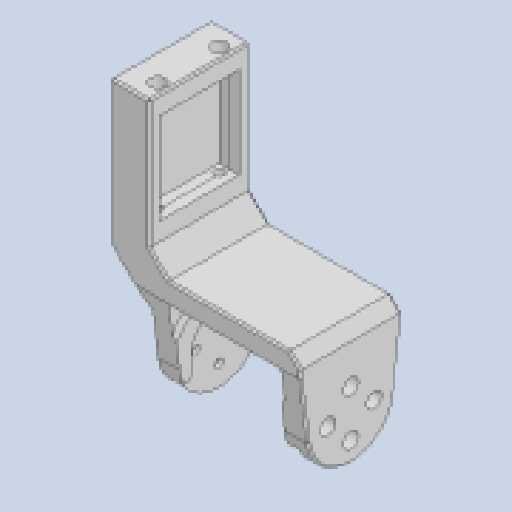
# Autodesk Inventor part: M-WristFlexion
Saved by Autodesk Inventor 2026 (Build 300175050, 175E)
## iProperties
Created: 2025-12-22
Part Number: M-WristFlexion
Material: Genérico
Document SubType Name: Modeling
Designer: user
Density: 1 g/cm^3
Appearance: Valor por defecto
Mass: 17.8828 g
Surface Area: 77.4828 cm^2
Volume: 17.8828 cm^3
Author: user
Autodesk Inventor part; units mm, degrees
ref_plane "YZ Plane" through (0, 0, 0) normal (1, 0, 0) x (0, 1, 0)
ref_plane "XZ Plane" through (0, 0, 0) normal (0, 1, 0) x (-1, 0, 0)
sketch "Boceto1" plane through (0, 0, 0) normal (0, 0, 1) x (1, 0, 0)
  line L0 (-14.6, -0.5214) -> (16.6711, -0.5214)
  line L1 (14.6, -5.5214) -> (-14.6, -5.5214)
  line L2 (14.6, -5.5214) -> (14.6, -32.4765)
  line L3 (14.6, -32.4765) -> (19.6, -32.4765)
  line L4 (19.6, -32.4765) -> (19.6, -3.4504)
  line L5 (-14.6, -5.5214) -> (-14.6, -32.4765)
  line L6 (-14.6, -32.4765) -> (-19.6, -32.4765)
  line L7 (-19.6, -32.4765) -> (-19.6, -9.6636)
  line L8 (-24.6, 9.3786) -> (-24.6, 32.5786)
  line L9 (-29.6, 37.5786) -> (-29.6, 0.3364)
  line L10 (-29.6, 0.3364) -> (-19.6, -9.6636)
  line L11 (16.6711, -0.5214) -> (19.6, -3.4504)
  line L12 (-24.6, 9.3786) -> (-19.6, 9.3786)
  line L13 (-19.6, 9.3786) -> (-19.6, 4.4786)
  line L14 (-24.5, 9.4786) -> (-24.5, 32.4786) construction
  line L15 (12.5, -5.5214) -> (-12.5, -5.5214)
  line L16 (14.5, -9.9753) -> (14.5, -20.9862)
  line L17 (-14.5, -9.9753) -> (-14.5, -20.9862)
  line L18 (11.8, -27.4765) -> (14.3, -27.4765)
  line L19 (-22.5, 32.4786) -> (-20.5, 32.4786) construction
  line L20 (-24.6, 32.5786) -> (-19.6, 32.5786)
  line L21 (-19.6, 32.5786) -> (-19.6, 37.5786)
  line L22 (-19.6, 37.5786) -> (-29.6, 37.5786)
  line L23 (-23.4172, 9.4786) -> (-14.45, 9.4786) construction
  line L24 (18.1355, -1.9859) -> (14.6, -5.5214) construction
  line L25 (-14.6, -0.5214) -> (-19.6, 4.4786)
  line L26 (-19.6, 32.5786) -> (-19.6, 9.3786)
  point P0 (0, 0)
  point P1 (19.6, -0.5214)
  point P2 (-19.6, -0.5214)
  point P3 (-14.5, -12.7214)
extrude "Extrusión1" add sketch "Boceto1" along normal mid plane 20.2 contours L0 L11 L4 L3 L2 L1 L5 L6 L7 L10 L9 L22 L21 L20 L8 L12 L13 L25
sketch "Boceto7" plane through (0, 0, -10.1) normal (0, 0, -1) x (-1, 0, 0)
  line L0 (19.6, 32.5786) -> (24.6, 32.5786) projected
  line L1 (24.6, 32.5786) -> (24.6, 9.3786) projected
  line L2 (24.6, 9.3786) -> (19.6, 9.3786) projected
  line L3 (19.6, 9.3786) -> (19.6, 4.4786) projected
  line L4 (19.6, 4.4786) -> (14.6, -0.5214) projected
  line L5 (14.6, -0.5214) -> (-16.6711, -0.5214) projected
  line L6 (-16.6711, -0.5214) -> (-19.6, -3.4504) projected
  line L7 (-19.6, -3.4504) -> (-19.6, -32.4765) projected
  line L8 (-19.6, -32.4765) -> (-14.6, -32.4765) projected
  line L9 (-14.6, -32.4765) -> (-14.6, -5.5214) projected
  line L10 (-14.6, -5.5214) -> (14.6, -5.5214) projected
  line L11 (14.6, -5.5214) -> (14.6, -32.4765) projected
  line L12 (14.6, -32.4765) -> (19.6, -32.4765) projected
  line L13 (19.6, -32.4765) -> (19.6, -9.6636) projected
  line L14 (19.6, -9.6636) -> (29.6, 0.3364) projected
  line L15 (29.6, 0.3364) -> (29.6, 37.5786) projected
  line L16 (29.6, 37.5786) -> (19.6, 37.5786) projected
  line L17 (19.6, 37.5786) -> (19.6, 32.5786) projected
  line L18 (19.6, 32.5786) -> (19.6, 9.3786)
  point P0 (0, 0)
  constraints: 2 end point, 1 collinear
extrude "Extrusión7" add sketch "Boceto7" along normal blind 3
mirror "Simetría2" about plane through (0, 0, 0) normal (0, 0, 1) of "Extrusión7"
sketch "Boceto8" plane through (-24.6, 32.5786, -10.1) normal (0, -1, 0) x (1, 0, 0)
  circle A0 centre (2.1, 18.1) radius 1 construction
  circle A1 centre (2.1, 18.1) radius 1.2
  circle A2 centre (2.1, 2.1) radius 1 construction
  circle A3 centre (2.1, 2.1) radius 1.2
  circle A4 centre (2.1, 2.1) radius 2
  circle A5 centre (2.1, 18.1) radius 2
  point P0 (24.6, 10.1)
  dimension "d70" = 0.2
  dimension "d71" = 0.2
  dimension "d72" = 4
  dimension "d73" = 4
  constraints: 4 centre point, 2 coincident
  measures "d70" radial gap between concentric circles of A0 A1
  measures "d71" radial gap between concentric circles of A2 A3
  measures "d72" diameter of A4
  measures "d73" diameter of A5
extrude "Extrusión8" cut sketch "Boceto8" along normal through all both and the other way through all contours A1 | A3
sketch "Boceto9" plane through (-24.6, 32.5786, -10.1) normal (0, -1, 0) x (1, 0, 0)
  circle A0 centre (2.1, 18.1) radius 1.2 construction
  circle A1 centre (2.1, 2.1) radius 1.2 construction
  line L0 (5, 0) -> (5, 20.2) construction
  line L1 (0, 20.2) -> (5, 20.2) construction
  line L2 (0, 20.2) -> (0, 0) construction
  line L3 (5, 0) -> (0, 0) construction
  circle A2 centre (2.1, 18.1) radius 2
  circle A3 centre (2.1, 2.1) radius 2
  point P0 (24.6, 10.1)
  dimension "d76" = 4
  dimension "d77" = 4
  constraints: 2 centre point, 2 coincident
  measures "d76" diameter of A2
  measures "d77" diameter of A3
extrude "Extrusión9" cut sketch "Boceto9" along normal blind 2.8 from surface at -5
extrude "Extrusión10" cut sketch "Boceto9" against normal blind 39.655 from surface at 65.0551
chamfer "Chaflán1" distance 0.2 distance2 2.5 4 edges at (-19.6, 9.3786, 0) (-19.6, 20.9786, 10.1) (-19.6, 32.5786, 0) (-19.6, 20.9786, -10.1)
sketch "Boceto10" plane through (14.6, -32.4765, -13.1) normal (-1, 0, 0) x (0, 0, 1)
  line L0 (0, 0) -> (26.2, 0) projected
  line L1 (26.2, 0) -> (26.2, 26.9551) projected
  line L2 (0, 26.9551) -> (26.2, 26.9551) projected
  line L3 (0, 0) -> (0, 26.9551) projected
  circle A0 centre (13.1, 12.9551) radius 8.2
  circle A1 centre (13.1, 12.9551) radius 11.2
  line L4 (26.2, 26.9551) -> (24.2078, 11.5213)
  line L5 (0, 26.9551) -> (1.9922, 11.5213)
  arc A2 (5.2352, 11.4903) -> (20.9648, 11.4903) centre (13.1, 12.9551) ccw construction
  arc A3 (12.9001, 20.7525) -> (12.2709, 5.1993) centre (13.1, 12.9551) ccw construction
  line L6 (13.1, 20.7551) -> (12.9, 20.7551) construction
  arc A4 (13.9291, 5.1993) -> (13.1, 20.7551) centre (13.1, 12.9551) ccw construction
  line L7 (13.6304, 5.1717) -> (13.9292, 5.1978) construction
  arc A5 (12.5697, 5.1731) -> (13.6303, 5.1731) centre (13.1, 12.9551) ccw construction
  line L8 (12.2708, 5.1978) -> (12.5696, 5.1717) construction
  circle A6 centre (13.1, 12.9551) radius 3 construction
  circle A7 centre (13.1, 6.9551) radius 0.8 construction
  circle A8 centre (19.1, 12.9551) radius 0.8 construction
  circle A9 centre (13.1, 18.9551) radius 0.8 construction
  circle A10 centre (7.1, 12.9551) radius 0.8 construction
  circle A11 centre (13.1, 6.9551) radius 1.1
  circle A12 centre (19.1, 12.9551) radius 1.1
  circle A13 centre (13.1, 18.9551) radius 1.1
  circle A14 centre (7.1, 12.9551) radius 1.1
  point P0 (13.1, 32.4765)
  dimension "d94" = 3
  dimension "d102" = 0.2
  dimension "d103" = 2.2
  dimension "d106" = 360
  constraints: 6 centre point, 4 end point, 2 coincident, 2 point on circle, 2 tangent, 9 other
  measures "d94" radial gap between concentric circles of A0 A1
  measures "d102" radial gap between concentric circles of A2 A0
  measures "d103" diameter of A11
extrude "Extrusión11" cut sketch "Boceto10" along normal through all both and the other way through all contours L3 L5 A1 L4 L1 L0 | A11 | A12 | A13 | A14
sketch "Boceto11" plane through (14.6, -19.5214, 0) normal (-1, 0, 0) x (0, 0, 1)
  line L0 (11.1078, -1.4338) -> (13.1, 14) projected
  line L1 (-13.1, 14) -> (13.1, 14) projected
  line L2 (-13.1, 14) -> (-11.1078, -1.4338) projected
  arc A0 (-11.1078, -1.4338) -> (11.1078, -1.4338) centre (0, 0) ccw projected
  circle A1 centre (-6, 0) radius 1.1 projected
  circle A2 centre (0, 6) radius 1.1 projected
  circle A3 centre (0, -6) radius 1.1 projected
  circle A4 centre (6, 0) radius 1.1 projected
  circle A5 centre (0, -6) radius 2
  arc A6 (-11.1078, -1.4338) -> (11.1078, -1.4338) centre (0, 0) ccw projected
  line L3 (-13.1, 14) -> (-11.1078, -1.4338) projected
  circle A7 centre (0, 0) radius 11.2
  circle A8 centre (0, 0) radius 8.2
  circle A9 centre (6, 0) radius 2
  circle A10 centre (0, 6) radius 2
  circle A11 centre (-6, 0) radius 2
  point P0 (0, 19.5214)
  point P1 (11.1078, -1.4338)
  dimension "d108" = 4
  dimension "d109" = 3
  dimension "d112" = 360
  constraints: 5 centre point, 2 coincident, 12 other
  measures "d108" diameter of A5
extrude "Extrusión12" add sketch "Boceto11" along normal blind 2.5 contours A0 A7
extrude "Extrusión13" cut sketch "Boceto11" along normal blind 3.8 from surface at -5 contours A1 | A2 | A3 | A4 | A5 | A9 | A10 | A11
chamfer "Chaflán3" distance 0.1 distance2 2 1 edges at (12.1, -19.5214, -8.2) measured on face at (12.1, -19.5214, -8.7)
chamfer "Chaflán4" distance 2.5 angle 45 1 edges at (14.6, -8.3214, 0)
extrude "Extrusión14" add sketch "Boceto11" against normal blind 2.5 from surface at 29.2 contours A0 A7
extrude "Extrusión15" cut sketch "Boceto11" against normal blind 3.8 from surface at 34.2 contours A1 | A2 | A3 | A4 | A5 | A9 | A10 | A11
chamfer "Chaflán5" distance 2 distance2 0.1 1 edges at (-12.1, -19.5214, -8.2) measured on face at (-12.6, -19.5214, -8.2)
chamfer "Chaflán6" distance 2.5 angle 45 1 edges at (-14.6, -8.3214, 0)
chamfer "Chaflán7" distance 0.5 angle 45 26 edges at (-19.6, 37.5786, 0) (-24.6, 37.5786, -13.1) (-19.6, 21.0286, -13.1) (-29.6, 18.9575, -13.1) (-29.6, 37.5786, 0) (-24.6, 37.5786, 13.1) (-29.6, 18.9575, 13.1) (-26.6711, -2.5925, -13.1) (-26.6711, -2.5925, 13.1) (-21.6711, -7.5925, 12.8327) (-19.6, 21.0286, 13.1) (-17.1, 1.9786, 13.1) (1.0355, -0.5214, 13.1) (18.1355, -1.9859, 13.1) (-19.6, -15.3094, 11.8366) (-19.6, -30.7214, 0) (-19.6, -15.3094, -11.8366) (-21.6711, -7.5925, -12.8327) (-17.1, 1.9786, -13.1) (1.0355, -0.5214, -13.1) (18.1355, -1.9859, -13.1) (19.6, -13.2383, -12.1039) (19.6, -30.7214, 0) (19.6, -13.2383, 12.1039) (19.6, -4.4859, -13.1) (19.6, -4.4859, 13.1)
sketch "Boceto12" plane through (-12.1, -19.5214, 0) normal (1, 0, 0) x (0, 0, -1)
  arc A0 (11.1078, -1.4338) -> (-11.1078, -1.4338) centre (0, 0) ccw projected
  arc A1 (-11.1078, -1.4338) -> (11.1078, -1.4338) centre (0, 0) ccw projected
  circle A2 centre (0, 0) radius 8.3 projected
  line L0 (-12.1179, 6.3912) -> (-11.1078, -1.4338) projected
  arc A3 (11.1078, -1.4338) -> (-11.1078, -1.4338) centre (0, 0) ccw projected
  line L1 (11.1078, -1.4338) -> (12.1179, 6.3912) projected
  arc A4 (12.1179, 6.3912) -> (-12.1179, 6.3912) centre (0, 0) ccw projected
  circle A5 centre (0, 0) radius 8.3 projected
  line L2 (-8.3, 0) -> (-8.3, -7.52)
  line L3 (8.3, 0) -> (8.3, -7.52)
  line L4 (12.5917, 10.0621) -> (11.1078, -1.4338) projected
  point P0 (0, 19.5214)
  point P1 (11.1078, -1.4338)
  point P2 (8.028, -2.1076)
  constraints: 4 end point, 3 horizontal alignment, 2 point on circle, 2 vertical, 4 other
extrude "Extrusión16" cut sketch "Boceto12" against normal blind 1.5
extrude "Extrusión17" cut sketch "Boceto12" along normal blind 1.5 from surface at 24.2
extrude "Extrusión18" cut sketch "Boceto12" against normal blind 2.5 contours A1 L2 A2 L3 | A2
extrude "Extrusión19" cut sketch "Boceto12" along normal blind 1 from surface at 25.7 contours A1 L2 A2 L3 | A2
fillet "Empalme1" radius 1 3 edges at (-14.1, -27.0414, -8.3) (-14.1, -27.0414, 8.3) (14.1, -27.0414, 8.3)
ref_plane "Plano de trabajo1" through (-14.6, -5.5214, 8) normal (0, 0, 1) x (1, 0, 0)
sketch "Boceto13" plane through (-29.6, 0.3364, 8) normal (0, 0, 1) x (1, 0, 0)
  line L0 (49.2, -19.8579) -> (49.2, -26.9635) projected
  line L1 (48.7, -27.6962) -> (44.2, -27.6962) projected
  line L2 (44.2, -27.6962) -> (44.2, -17.6465) projected
  line L3 (10, -26.9635) -> (10, -19.8579) projected
  line L4 (15, -17.6465) -> (15, -27.6962) projected
  line L5 (15, -27.6962) -> (10.5, -27.6962) projected
  line L6 (9.5, 37.2421) -> (10, 36.7421) projected
  line L7 (10, 36.7421) -> (10, 32.4421) projected
  line L8 (10, 32.4421) -> (8.3, 32.3061) projected
  line L9 (5.9, 32.2421) -> (5, 32.2421) projected
  line L10 (5, 32.2421) -> (5, 9.0421) projected
  line L11 (5, 9.0421) -> (5.9, 9.0421) projected
  line L12 (8.3, 8.9781) -> (10, 8.8421) projected
  line L13 (10, 8.8421) -> (10, 4.1421) projected
  line L14 (10, 4.1421) -> (15, -0.8579) projected
  line L15 (15, -0.8579) -> (46.2711, -0.8579) projected
  line L16 (46.2711, -0.8579) -> (49.2, -3.7868) projected
  line L17 (49.2, -3.7868) -> (49.2, -19.8579) projected
  line L18 (44.2, -17.6465) -> (43.2, -17.6465) projected
  line L19 (43.2, -17.6465) -> (43.2, -9.9943) projected
  line L20 (44.2, -8.7363) -> (44.2, -5.8579) projected
  line L21 (44.2, -5.8579) -> (15, -5.8579) projected
  line L22 (15, -5.8579) -> (15, -8.7363) projected
  line L23 (16, -9.9943) -> (16, -17.6465) projected
  line L24 (16, -17.6465) -> (15, -17.6465) projected
  line L25 (10, -19.8579) -> (10, -10) projected
  line L26 (10, -10) -> (9.1, -9.1) projected
  line L27 (0, 0) -> (0, 36.7421) projected
  line L28 (0, 36.7421) -> (0.5, 37.2421) projected
  line L29 (9.1, 37.2421) -> (9.5, 37.2421) projected
  line L30 (9.1, 6.8421) -> (0, 6.8421)
  line L31 (9.1, 6.8421) -> (9.1, -9.1)
  line L32 (8.3, 6.8421) -> (5.9, 6.8421) projected
  line L33 (9.1, 6.8421) -> (5.1, 6.8421) projected
  line L34 (9.1, -9.1) -> (9.1, 6.8421) projected
  line L35 (9.1, 6.8421) -> (8.3, 6.8421) projected
  line L36 (8.3, 6.8421) -> (8.3, 8.9781) projected
  line L37 (45.4, -19.8579) -> (49.2, -19.8579) projected
  line L38 (13.8, -19.8579) -> (10, -19.8579) projected
  line L39 (8.3, 32.3061) -> (8.3, 34.4421) projected
  line L40 (8.3, 34.4421) -> (9.1, 34.4421) projected
  line L41 (9.1, 34.4421) -> (9.1, 37.2421) projected
  line L42 (5.9, 9.0421) -> (5.9, 6.8421) projected
  line L43 (5.9, 6.8421) -> (5.1, 6.8421) projected
  line L44 (5.1, 6.8421) -> (5.1, -5.1) projected
  line L45 (5.1, -5.1) -> (0, 0) projected
  line L46 (0.5, 37.2421) -> (5.1, 37.2421) projected
  line L47 (5.1, 37.2421) -> (5.1, 34.4421) projected
  line L48 (5.1, 34.4421) -> (5.9, 34.4421) projected
  line L49 (5.9, 34.4421) -> (5.9, 32.2421) projected
  line L50 (9.1, -9.1) -> (5.1, -5.1) projected
  line L51 (5.1, -5.1) -> (9.1, -9.1)
  line L52 (5.1, 4.8421) -> (0, 4.8421)
  line L53 (5.1, 4.8421) -> (9.1, 4.8421)
  point P0 (29.6, -0.3364)
  point P1 (5.1, 6.8421)
  point P2 (9.1, 4.8421)
  dimension "d147" = 2
  constraints: 11 end point, 5 point on line, 4 perpendicular, 2 collinear, 2 parallel, 4 other
  measures "d147" distance between parallel lines of L52 L30
extrude "Extrusión20" cut sketch "Boceto13" along normal mid plane 4 contours L53 L31 L50 L44 | L44 L45 L27 L52
chamfer "Chaflán8" distance 2 distance2 9.1 2 edges at (-29.6, 2.7575, 10) (-29.6, 2.7575, 6)
sketch "Boceto14" plane through (-22.5, 5.1785, 8) normal (0, -1, 0) x (1, 0, 0)
  circle A0 centre (0, 0) radius 2 projected
  line L0 (2, 0) -> (2, 2) projected
  line L1 (2, 2) -> (-7.1, 4) projected
  line L2 (-7.1, 4) -> (-7.1, -4) projected
  line L3 (2, -2) -> (-7.1, -4) projected
  line L4 (2, -2) -> (2, 0) projected
  line L5 (0, 0) -> (-7.1, 0) construction
  line L6 (-7.1, -20.6) -> (-7.1, 4.6) projected
  line L7 (-1.9365, 0.5) -> (-7.1, 0.5)
  line L8 (-1.9365, -0.5) -> (-7.1, -0.5)
  circle A1 centre (0, 0) radius 2 projected
  point P0 (22.5, -8)
  point P1 (-1.9365, -0.5)
  dimension "d155" = 1
  constraints: 6 end point, 3 point on line, 2 parallel, 2 point on circle, 1 perpendicular, 1 other
  measures "d155" distance between parallel lines of L8 L7
extrude "Extrusión22" cut sketch "Boceto14" against normal blind 1.5 contours A0 L8 L2 L7
chamfer "Chaflán9" distance 1.5 angle 45 2 edges at (-27.0182, 5.1785, 8.5) (-27.0182, 5.1785, 7.5)
mirror "Simetría3" about plane through (0, 0, 0) normal (0, 0, 1) of "Extrusión20", "Chaflán8", "Extrusión22", "Chaflán9"
equation "\"d48\" = d47"
equation "\"d47\" = 2.928932"
